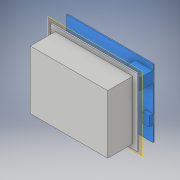
# Autodesk Inventor part: Arduino
Saved by Autodesk Inventor 2019 (Build 230136000, 136)
## iProperties
Created: 2018-12-25
Part Number: Arduino
Material: Generic
Document SubType Name: Modeling
Designer: Martin
Density: 1 g/cm^3
Appearance: Default
Author: Martin
Autodesk Inventor part; units mm, degrees
ref_plane "YZ Plane" through (0, 0, 0) normal (1, 0, 0) x (0, 1, 0)
ref_plane "XZ Plane" through (0, 0, 0) normal (0, 1, 0) x (-1, 0, 0)
ref_plane "XY Plane" through (0, 0, 0) normal (0, 0, 1) x (1, 0, 0)
sketch "Sketch1" plane through (0, 0, 0) normal (0, 0, 1) x (1, 0, 0)
  line L0 (-34.5, 27) -> (34.5, 27)
  line L1 (34.5, 27) -> (34.5, -27)
  line L2 (34.5, -27) -> (-34.5, -27)
  line L3 (-34.5, -27) -> (-34.5, 27)
  line L4 (-34.5, 27) -> (34.5, -27) construction
  line L5 (34.5, 27) -> (-34.5, -27) construction
  point P0 (0, 0)
  dimension "d0" = 69
  dimension "d1" = 54
  constraints: 12 end point, 2 midpoint, 2 parallel, 1 horizontal, 1 perpendicular
  measures "d0" distance of L1.end L2.end
  measures "d1" distance of L0.end L1.end
extrude "Extrusion1" add sketch "Sketch1" along normal blind 1
sketch "Sketch2" plane through (0, 0, 1) normal (0, 0, 1) x (1, 0, 0)
  line L0 (34.5, 23) -> (20.5, 23)
  line L1 (20.5, 23) -> (20.5, 14.15)
  line L2 (20.5, 14.15) -> (34.5, 14.15)
  line L3 (34.5, 14.15) -> (34.5, 23)
  line L4 (28.8, -7.1) -> (34.5, -7.1)
  line L5 (34.5, -7.1) -> (34.5, -14.7)
  line L6 (34.5, -14.7) -> (28.8, -14.7)
  line L7 (28.8, -14.7) -> (28.8, -7.1)
  line L8 (34.5, -27) -> (34.5, 27) projected
  line L9 (34.5, 27) -> (-34.5, 27) projected
  line L10 (-34.5, -27) -> (34.5, -27) projected
  point P0 (0, 0)
  dimension "d4" = 8.85
  dimension "d5" = 14
  dimension "d6" = 4
  dimension "d7" = 7.6
  dimension "d8" = 5.7
  dimension "d9" = 12.3
  constraints: 16 end point, 4 parallel, 2 horizontal, 2 perpendicular, 1 collinear
  measures "d4" distance of L2.end L0.start
  measures "d5" distance of L0.start L0.end
  measures "d6" distance between parallel lines of L0 L9
  measures "d7" distance of L4.end L5.end
  measures "d8" distance of L4.start L4.end
  measures "d9" distance between parallel lines of L10 L6
extrude "Extrusion2" add sketch "Sketch2" along normal blind 10.5 contours L3 L2 L1 L0
extrude "Extrusion3" add sketch "Sketch2" along normal blind 3 contours L5 L6 L7 L4
ref_plane "Work Plane1" through (0, 0, 12.5) normal (0, 0, 1) x (1, 0, 0)
sketch "Sketch3" plane through (0, 0, 12.5) normal (0, 0, 1) x (1, 0, 0)
  line L0 (-34.5, 27) -> (34.5, 27) projected
  line L1 (-34.5, -27) -> (34.5, -27) projected
  line L2 (34.5, 27) -> (-34.5, 27)
  line L3 (-34.5, 27) -> (-34.5, -27)
  line L4 (-34.5, -27) -> (34.5, -27)
  line L5 (34.5, -27) -> (34.5, 27)
  point P0 (0, 0)
  constraints: 8 end point, 2 parallel, 1 horizontal, 1 perpendicular
extrude "Extrusion4" add sketch "Sketch3" along normal blind 1
sketch "Sketch4" plane through (0, 0, 13.5) normal (0, 0, 1) x (1, 0, 0)
  line L0 (-34.5, -27) -> (34.5, -27) projected
  line L1 (34.5, 27) -> (-34.5, 27)
  line L2 (-34.5, 27) -> (-34.5, -27)
  line L3 (-34.5, -27) -> (34.5, -27)
  line L4 (34.5, -27) -> (34.5, 27)
  line L5 (30.8377, 23.3377) -> (-30.8377, 23.3377)
  line L6 (-30.8377, 23.3377) -> (-30.8377, -23.3377)
  line L7 (-30.8377, -23.3377) -> (30.8377, -23.3377)
  line L8 (30.8377, -23.3377) -> (30.8377, 23.3377)
  point P0 (0, 0)
  constraints: 16 end point, 4 parallel, 2 perpendicular, 1 horizontal
extrude "Extrusion5" add sketch "Sketch4" along normal blind 20 contours L8 L7 L6 L5
body "Solid1"
